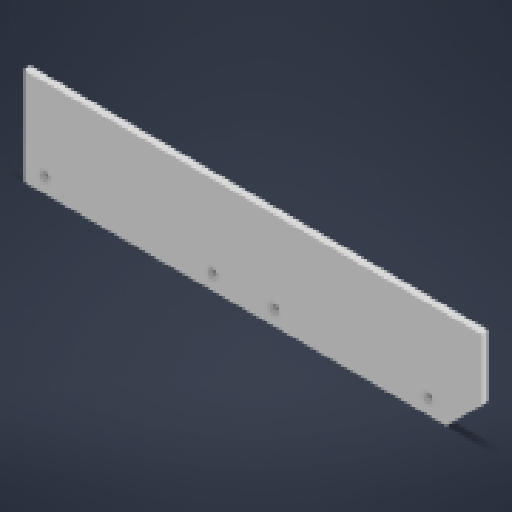
# Autodesk Inventor part: ФАЛЬШБОРТА
Saved by Autodesk Inventor 2025 (Build 290162000, 162)
## iProperties
Created: 2025-01-26
Part Number: ФАЛЬШБОРТА
Material: Типовые
Document SubType Name: Modeling
Designer: GameHD
Density: 1 g/cm^3
Appearance: По умолчанию
Author: GameHD
Autodesk Inventor part; units mm, degrees
ref_plane "YZ Plane" through (0, 0, 0) normal (1, 0, 0) x (0, 1, 0)
ref_plane "XZ Plane" through (0, 0, 0) normal (0, 1, 0) x (-1, 0, 0)
ref_plane "XY Plane" through (0, 0, 0) normal (0, 0, 1) x (1, 0, 0)
sketch "Эскиз1" plane through (0, 0, 0) normal (0, 0, 1) x (1, 0, 0)
  line L0 (0, 0) -> (260, 0)
  line L1 (260, 0) -> (260, 55)
  line L2 (260, 55) -> (0, 55)
  line L3 (0, 55) -> (0, 0)
  dimension "d0" = 260
  dimension "d1" = 55
  constraints: 8 end point, 2 parallel, 1 horizontal, 1 perpendicular
  measures "d0" distance of L2.end L1.end
  measures "d1" distance of L1.end L0.end
extrude "Выдавливание1" add sketch "Эскиз1" along normal blind 4
sketch "Эскиз2" plane through (0, 0, 4) normal (0, 0, 1) x (1, 0, 0)
  line L0 (260, 55) -> (0, 55) projected
  line L1 (260, 55) -> (260, 35)
  line L2 (260, 0) -> (260, 55) projected
  line L3 (260, 55) -> (240, 55)
  line L4 (240, 55) -> (260, 35)
  line L5 (260, 27.5) -> (225.425, 27.5)
  line L6 (260, 0) -> (260, 20)
  line L7 (260, 0) -> (240, 0)
  line L8 (240, 0) -> (260, 20)
  point P0 (0, 0)
  dimension "d4" = 20
  dimension "d5" = 20
  constraints: 14 end point, 2 point on line, 2 symmetric about line, 1 horizontal, 1 midpoint
  measures "d4" distance of L0.start L1.end
  measures "d5" distance of L0.start L3.end
extrude "Выдавливание2" cut sketch "Эскиз2" against normal blind 4 contours L7 L8 L2
sketch "Эскиз3" plane through (0, 0, 0) normal (0, 0, -1) x (-1, 0, 0)
  line L0 (6.1414, 6.05) -> (-239.9996, 6.05) projected
  line L1 (6.1414, 12.1816) -> (-239.9996, 12.1816) projected
  line L2 (-7.1405, 6.05) -> (-7.1405, 12.1816)
  line L3 (-7.1405, 9.1158) -> (-109.5375, 9.1158)
  circle A0 centre (-12.7, 9.1158) radius 2.1
  circle A1 centre (-230.1875, 9.1158) radius 2.1
  circle A2 centre (-107.95, 9.1158) radius 2.1
  circle A3 centre (-142.875, 9.1158) radius 2.1
  point P0 (0, 0)
  dimension "d8" = 4.2
  dimension "d9" = 4.2
  dimension "d10" = 4.2
  dimension "d11" = 4.2
  constraints: 5 point on line, 4 centre point, 4 end point, 1 midpoint, 1 parallel, 1 perpendicular
  measures "d8" diameter of A0
  measures "d9" diameter of A1
  measures "d10" diameter of A2
  measures "d11" diameter of A3
extrude "Выдавливание3" cut sketch "Эскиз3" against normal blind 4.2
equation "\"d12\" = d9"
